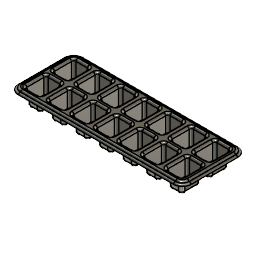
Day5IceTray (Autodesk Fusion 360 design; units mm, degrees)
part number: 2025-11-22-08-57-42-411
Autodesk Fusion 360 part; units mm, degrees
sketch "Sketch1" plane through (0, 0, 0) normal (0, 0, 1) x (1, 0, 0)
  line L0 (0, 0) -> (300, 0)
  line L1 (300, 0) -> (300, 104)
  line L2 (300, 104) -> (0, 104)
  line L3 (0, 104) -> (0, 0)
  dimension "d1" = 300
  dimension "d2" = 104
  constraint horizontal L0
  constraint vertical L1
  constraint horizontal L2
  constraint vertical L3
  constraint coincident L0.start L3.end
  measures "d1" distance of L0.start L0.end
  measures "d2" distance of L0.start L2.end
extrude "Extrude1" add sketch "Sketch1" along normal blind 50
sketch "Sketch2" plane through (0, 0, 50) normal (0, 0, 1) x (-1, 0, 0)
  line L0 (0, -104) -> (0, 0)
  line L1 (0, 0) -> (-300, 0)
  line L2 (-300, 0) -> (-300, -104)
  line L3 (-300, -104) -> (0, -104)
  line L4 (-7, -97) -> (-37, -97)
  line L5 (-37, -97) -> (-37, -57)
  line L6 (-37, -57) -> (-7, -57)
  line L7 (-7, -57) -> (-7, -97)
  dimension "d5" = 30
  dimension "d6" = 40
  dimension "d7" = 7
  dimension "d8" = 7
  constraint horizontal L4
  constraint vertical L5
  constraint horizontal L6
  constraint vertical L7
  measures "d5" distance of L4.start L4.end
  measures "d6" distance of L4.start L6.end
  measures "d7" distance of L0 L7
  measures "d8" distance of L3 L4
extrude "Extrude2" cut sketch "Sketch2" against normal blind 30 draft -10 contours L4 L5 L6 L7
fillet "Fillet1" radius 4 4 faces at (8.7633, 72.0966, 40) (18.7633, 95.2367, 40) (35.2367, 81.9034, 40) (25.2367, 58.7633, 40)
pattern_linear "R-Pattern1" count 2 spacing 50 along (0, -1, 0) count 7 spacing 42.5 along (1, 0, 0) of "Extrude2", "Fillet1"
shell "Shell1" thickness 2 removed faces 5 at (200, 104, 16.6667) at (300, 34.6667, 16.6667) at (100, 0, 16.6667) at (0, 69.3333, 16.6667) at (100, 69.3333, 0)
fillet "Fillet2" radius 10 1 edges at (300, 0, 49)
fillet "Fillet3" radius 10 1 edges at (0, 0, 49)
fillet "Fillet4" radius 10 1 edges at (0, 104, 49)
fillet "Fillet5" radius 10 1 edges at (300, 104, 49)
ref_plane "WorkPlane1" through (150, 52, 49) normal (0, 1, 0) x (-1, 0, 0)
sketch "Sketch3" plane through (0, 52, 0) normal (0, 1, 0) x (1, 0, 0)
  line L0 (0, -50) -> (0, -45)
  line L1 (0, -45) -> (-6.2173, -45)
  line L2 (-6.2173, -45) -> (-6.2173, -47.5)
  line L3 (-6.2173, -47.5) -> (-2.2097, -47.5)
  line L4 (-2.2097, -47.5) -> (-2.2097, -50)
  line L5 (-2.2097, -50) -> (0, -50)
  dimension "d26" = 2.2097
  constraint vertical L0
  constraint perpendicular L0 L1
  constraint perpendicular L1 L2
  constraint perpendicular L2 L3
  constraint perpendicular L3 L4
  constraint perpendicular L0 L5
  measures "d26" distance of L0.start L4.end
sweep "Sweep1" add profiles "Sketch3" along 8 edges at (300, 52, 50) (297.0711, 101.0711, 50) (150, 104, 50) (2.9289, 101.0711, 50) (0, 52, 50) (2.9289, 2.9289, 50) (150, 0, 50) (297.0711, 2.9289, 50) section 1
fillet "Fillet6" radius 4 8 edges at (302.2097, 52, 50) (298.6335, 102.6335, 50) (150, 106.2097, 50) (1.3665, 102.6335, 50) (-2.2097, 52, 50) (1.3665, 1.3665, 50) (150, -2.2097, 50) (298.6335, 1.3665, 50)
fillet "Fillet7" radius 4 8 edges at (306.2173, 52, 47.5) (301.4674, 105.4674, 47.5) (150, 110.2173, 47.5) (-1.4674, 105.4674, 47.5) (-6.2173, 52, 47.5) (-1.4674, -1.4674, 47.5) (150, -6.2173, 47.5) (301.4674, -1.4674, 47.5)
